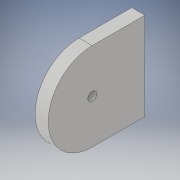
# Autodesk Inventor part: Part12
Saved by Autodesk Inventor 2019 (Build 230136000, 136)
## iProperties
Created: 2021-08-30
Part Number: Part12
Material: 一般
Document SubType Name: Sheet Metal
Designer: yuta
Density: 1 g/cm^3
Sheet Metal Rule: Default_mm
Appearance: 既定
Author: yuta
Autodesk Inventor part; units mm, degrees
ref_plane "YZ Plane" through (0, 0, 0) normal (1, 0, 0) x (0, 1, 0)
ref_plane "XZ Plane" through (0, 0, 0) normal (0, 1, 0) x (-1, 0, 0)
ref_plane "XY Plane" through (0, 0, 0) normal (0, 0, 1) x (1, 0, 0)
sketch "スケッチ1" plane through (0, 0, 0) normal (1, 0, 0) x (0, 1, 0)
  line L0 (7.2151, 11.0659) -> (-12.7849, 11.0659)
  line L1 (-12.7849, 11.0659) -> (-12.7849, -0.9341)
  line L2 (-12.7849, -0.9341) -> (7.2151, -0.9341)
  line L3 (7.2151, -0.9341) -> (7.2151, 11.0659)
  arc A0 (7.2151, 11.0659) -> (-12.7849, 11.0659) centre (-2.7849, 11.0659) ccw
  point P0 (0, 0)
  dimension "d0" = 20
  dimension "d1" = 12
  constraints: 8 end point, 2 parallel, 2 point on circle, 2 tangent, 1 centre point, 1 horizontal, 1 perpendicular
  measures "d0" distance of L2.end L1.end
  measures "d1" distance of L1.end L0.end
extrude "押し出し1" add sketch "スケッチ1" along normal blind 3
sketch "スケッチ2" plane through (3, 0, 0) normal (1, 0, 0) x (0, 0, -1)
  arc A0 (-11.0659, 7.2151) -> (-11.0659, -12.7849) centre (-11.0659, -2.7849) ccw projected
  circle A1 centre (-11.0659, -2.7849) radius 1
  point P0 (0, 0)
  dimension "d4" = 2
  constraints: 1 centre point, 1 coincident
  measures "d4" diameter of A1
hole "穴1" at (3, -2.7849, 11.0659) direction (-1, 0, 0) diameter 2 depth 10
equation "\"BendRadius\" = Thickness"
equation "\"BendReliefWidth\" = Thickness"
equation "\"BendReliefDepth\" = 0.5 * Thickness"
equation "\"CornerReliefSize\" = 4 * Thickness"
equation "\"MinimumRemnant\" = 2 * Thickness"
equation "\"TransitionRadius\" = BendRadius"
equation "\"JacobiRadiusSize\" = BendRadius"
equation "\"GapSize\" = Thickness"
equation "\"Thickness\" = 0.5"
